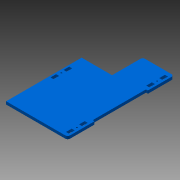
# Autodesk Inventor part: boardCaseBottom
Saved by Autodesk Inventor 2013 (Build 170138000, 138)
## iProperties
Created: 2015-01-14
Part Number: boardCaseBottom
Material: Generic
Document SubType Name: Modeling
Designer: dzban
Density: 1 g/cm^3
Author: dzban
Autodesk Inventor part; units mm, degrees
ref_plane "YZ Plane" through (0, 0, 0) normal (1, 0, 0) x (0, 1, 0)
ref_plane "XZ Plane" through (0, 0, 0) normal (0, 1, 0) x (-1, 0, 0)
ref_plane "XY Plane" through (0, 0, 0) normal (0, 0, 1) x (1, 0, 0)
sketch "Sketch1" plane through (0, 0, 0) normal (0, 0, 1) x (1, 0, 0)
  line L0 (-4.2207, 7.2045) -> (-10.6207, 7.2045)
  line L1 (-10.6207, 7.2045) -> (-10.6207, 19.2045)
  line L2 (-10.6207, 19.2045) -> (-4.2207, 19.2045)
  line L3 (-4.2207, 19.2045) -> (-4.2207, 7.2045)
  circle A0 centre (-7.4207, 27.0045) radius 1.5
  line L4 (-4.2207, 34.8045) -> (-10.6207, 34.8045)
  line L5 (-10.6207, 34.8045) -> (-10.6207, 46.8045)
  line L6 (-10.6207, 46.8045) -> (-4.2207, 46.8045)
  line L7 (-4.2207, 46.8045) -> (-4.2207, 34.8045)
  line L8 (-4.2207, 177.2045) -> (-10.6207, 177.2045)
  line L9 (-10.6207, 177.2045) -> (-10.6207, 189.2045)
  line L10 (-10.6207, 189.2045) -> (-4.2207, 189.2045)
  line L11 (-4.2207, 189.2045) -> (-4.2207, 177.2045)
  circle A1 centre (-7.4207, 197.0045) radius 1.5
  line L12 (-4.2207, 204.8045) -> (-10.6207, 204.8045)
  line L13 (-10.6207, 204.8045) -> (-10.6207, 216.8045)
  line L14 (-10.6207, 216.8045) -> (-4.2207, 216.8045)
  line L15 (-4.2207, 216.8045) -> (-4.2207, 204.8045)
  line L16 (-120.6567, 90.7) -> (-127.0567, 90.7)
  line L17 (-127.0567, 90.7) -> (-127.0567, 102.7)
  line L18 (-127.0567, 102.7) -> (-120.6567, 102.7)
  line L19 (-120.6567, 102.7) -> (-120.6567, 90.7)
  circle A2 centre (-123.8567, 110.5) radius 1.5
  line L20 (-120.6567, 118.3) -> (-127.0567, 118.3)
  line L21 (-127.0567, 118.3) -> (-127.0567, 130.3)
  line L22 (-127.0567, 130.3) -> (-120.6567, 130.3)
  line L23 (-120.6567, 130.3) -> (-120.6567, 118.3)
  line L24 (-66, 160) -> (-130.4, 160)
  line L25 (-130.4, 160) -> (-130.4, 0)
  line L26 (-130.4, 0) -> (-5, 0)
  arc A3 (-5, 0) -> (0, 5) centre (-5, 5) ccw
  line L27 (0, 5) -> (0, 56)
  arc A4 (0, 56) -> (-1, 57) centre (-1, 56) ccw
  line L28 (-1, 57) -> (-3, 57)
  arc A5 (-4, 58) -> (-3, 57) centre (-3, 58) ccw
  line L29 (-4, 58) -> (-4, 169)
  arc A6 (-3, 170) -> (-4, 169) centre (-3, 169) ccw
  line L30 (-3, 170) -> (-1, 170)
  arc A7 (-1, 170) -> (0, 171) centre (-1, 171) ccw
  line L31 (0, 171) -> (0, 220)
  arc A8 (0, 220) -> (-5, 225) centre (-5, 220) ccw
  line L32 (-5, 225) -> (-61, 225)
  arc A9 (-61, 225) -> (-66, 220) centre (-61, 220) ccw
  line L33 (-66, 220) -> (-66, 160)
  point P0 (0, 0)
  point P1 (0, 0)
  constraints: 68 end point, 14 point on circle, 10 centre point
extrude "Extrusion1" add sketch "Sketch1" along normal blind 6
body "Solid1"
